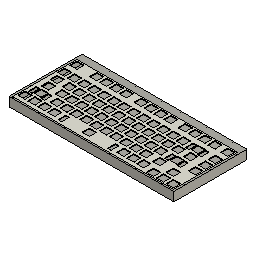
Keyboard_case (Autodesk Fusion 360 design; units mm, degrees)
part number: 2026-03-22-16-39-54-698
Autodesk Fusion 360 part; units mm, degrees
note: some values were not read from the file. Set by a fixed rule: which face or edge a step refers to.
(part 1 of 2)
sketch "plate-2026-03-22T13_27_17.077Z" plane through (0, 0, 0) normal (0, 0, 1) x (1, 0, 0)
  line L0 (3.025, -2.525) -> (16.025, -2.525)
  line L1 (3.025, -16.525) -> (16.025, -16.525)
  line L2 (2.525, -3.025) -> (2.525, -16.025)
  line L3 (16.525, -3.025) -> (16.525, -16.025)
  arc A0 (3.025, -2.525) -> (2.525, -3.025) centre (3.025, -3.025) ccw
  arc A1 (16.525, -3.025) -> (16.025, -2.525) centre (16.025, -3.025) ccw
  arc A2 (2.525, -16.025) -> (3.025, -16.525) centre (3.025, -16.025) ccw
  arc A3 (16.025, -16.525) -> (16.525, -16.025) centre (16.025, -16.025) ccw
  line L4 (41.125, -2.525) -> (54.125, -2.525)
  line L5 (41.125, -16.525) -> (54.125, -16.525)
  line L6 (40.625, -3.025) -> (40.625, -16.025)
  line L7 (54.625, -3.025) -> (54.625, -16.025)
  arc A4 (41.125, -2.525) -> (40.625, -3.025) centre (41.125, -3.025) ccw
  arc A5 (54.625, -3.025) -> (54.125, -2.525) centre (54.125, -3.025) ccw
  arc A6 (40.625, -16.025) -> (41.125, -16.525) centre (41.125, -16.025) ccw
  arc A7 (54.125, -16.525) -> (54.625, -16.025) centre (54.125, -16.025) ccw
  line L8 (60.175, -2.525) -> (73.175, -2.525)
  line L9 (60.175, -16.525) -> (73.175, -16.525)
  line L10 (59.675, -3.025) -> (59.675, -16.025)
  line L11 (73.675, -3.025) -> (73.675, -16.025)
  arc A8 (60.175, -2.525) -> (59.675, -3.025) centre (60.175, -3.025) ccw
  arc A9 (73.675, -3.025) -> (73.175, -2.525) centre (73.175, -3.025) ccw
  arc A10 (59.675, -16.025) -> (60.175, -16.525) centre (60.175, -16.025) ccw
  arc A11 (73.175, -16.525) -> (73.675, -16.025) centre (73.175, -16.025) ccw
  line L12 (79.225, -2.525) -> (92.225, -2.525)
  line L13 (79.225, -16.525) -> (92.225, -16.525)
  line L14 (78.725, -3.025) -> (78.725, -16.025)
  line L15 (92.725, -3.025) -> (92.725, -16.025)
  arc A12 (79.225, -2.525) -> (78.725, -3.025) centre (79.225, -3.025) ccw
  arc A13 (92.725, -3.025) -> (92.225, -2.525) centre (92.225, -3.025) ccw
  arc A14 (78.725, -16.025) -> (79.225, -16.525) centre (79.225, -16.025) ccw
  arc A15 (92.225, -16.525) -> (92.725, -16.025) centre (92.225, -16.025) ccw
  line L16 (98.275, -2.525) -> (111.275, -2.525)
  line L17 (98.275, -16.525) -> (111.275, -16.525)
  line L18 (97.775, -3.025) -> (97.775, -16.025)
  line L19 (111.775, -3.025) -> (111.775, -16.025)
  arc A16 (98.275, -2.525) -> (97.775, -3.025) centre (98.275, -3.025) ccw
  arc A17 (111.775, -3.025) -> (111.275, -2.525) centre (111.275, -3.025) ccw
  arc A18 (97.775, -16.025) -> (98.275, -16.525) centre (98.275, -16.025) ccw
  arc A19 (111.275, -16.525) -> (111.775, -16.025) centre (111.275, -16.025) ccw
  line L20 (126.85, -2.525) -> (139.85, -2.525)
  line L21 (126.85, -16.525) -> (139.85, -16.525)
  line L22 (126.35, -3.025) -> (126.35, -16.025)
  line L23 (140.35, -3.025) -> (140.35, -16.025)
  arc A20 (126.85, -2.525) -> (126.35, -3.025) centre (126.85, -3.025) ccw
  arc A21 (140.35, -3.025) -> (139.85, -2.525) centre (139.85, -3.025) ccw
  arc A22 (126.35, -16.025) -> (126.85, -16.525) centre (126.85, -16.025) ccw
  arc A23 (139.85, -16.525) -> (140.35, -16.025) centre (139.85, -16.025) ccw
  line L24 (145.9, -2.525) -> (158.9, -2.525)
  line L25 (145.9, -16.525) -> (158.9, -16.525)
  line L26 (145.4, -3.025) -> (145.4, -16.025)
  line L27 (159.4, -3.025) -> (159.4, -16.025)
  arc A24 (145.9, -2.525) -> (145.4, -3.025) centre (145.9, -3.025) ccw
  arc A25 (159.4, -3.025) -> (158.9, -2.525) centre (158.9, -3.025) ccw
  arc A26 (145.4, -16.025) -> (145.9, -16.525) centre (145.9, -16.025) ccw
  arc A27 (158.9, -16.525) -> (159.4, -16.025) centre (158.9, -16.025) ccw
  line L28 (164.95, -2.525) -> (177.95, -2.525)
  line L29 (164.95, -16.525) -> (177.95, -16.525)
  line L30 (164.45, -3.025) -> (164.45, -16.025)
  line L31 (178.45, -3.025) -> (178.45, -16.025)
  arc A28 (164.95, -2.525) -> (164.45, -3.025) centre (164.95, -3.025) ccw
  arc A29 (178.45, -3.025) -> (177.95, -2.525) centre (177.95, -3.025) ccw
  arc A30 (164.45, -16.025) -> (164.95, -16.525) centre (164.95, -16.025) ccw
  arc A31 (177.95, -16.525) -> (178.45, -16.025) centre (177.95, -16.025) ccw
  line L32 (184, -2.525) -> (197, -2.525)
  line L33 (184, -16.525) -> (197, -16.525)
  line L34 (183.5, -3.025) -> (183.5, -16.025)
  line L35 (197.5, -3.025) -> (197.5, -16.025)
  arc A32 (184, -2.525) -> (183.5, -3.025) centre (184, -3.025) ccw
  arc A33 (197.5, -3.025) -> (197, -2.525) centre (197, -3.025) ccw
  arc A34 (183.5, -16.025) -> (184, -16.525) centre (184, -16.025) ccw
  arc A35 (197, -16.525) -> (197.5, -16.025) centre (197, -16.025) ccw
  line L36 (211.6225, -2.525) -> (224.6225, -2.525)
  line L37 (211.6225, -16.525) -> (224.6225, -16.525)
  line L38 (211.1225, -3.025) -> (211.1225, -16.025)
  line L39 (225.1225, -3.025) -> (225.1225, -16.025)
  arc A36 (211.6225, -2.525) -> (211.1225, -3.025) centre (211.6225, -3.025) ccw
  arc A37 (225.1225, -3.025) -> (224.6225, -2.525) centre (224.6225, -3.025) ccw
  arc A38 (211.1225, -16.025) -> (211.6225, -16.525) centre (211.6225, -16.025) ccw
  arc A39 (224.6225, -16.525) -> (225.1225, -16.025) centre (224.6225, -16.025) ccw
  line L40 (230.6725, -2.525) -> (243.6725, -2.525)
  line L41 (230.6725, -16.525) -> (243.6725, -16.525)
  line L42 (230.1725, -3.025) -> (230.1725, -16.025)
  line L43 (244.1725, -3.025) -> (244.1725, -16.025)
  arc A40 (230.6725, -2.525) -> (230.1725, -3.025) centre (230.6725, -3.025) ccw
  arc A41 (244.1725, -3.025) -> (243.6725, -2.525) centre (243.6725, -3.025) ccw
  arc A42 (230.1725, -16.025) -> (230.6725, -16.525) centre (230.6725, -16.025) ccw
  arc A43 (243.6725, -16.525) -> (244.1725, -16.025) centre (243.6725, -16.025) ccw
  line L44 (249.7225, -2.525) -> (262.7225, -2.525)
  line L45 (249.7225, -16.525) -> (262.7225, -16.525)
  line L46 (249.2225, -3.025) -> (249.2225, -16.025)
  line L47 (263.2225, -3.025) -> (263.2225, -16.025)
  arc A44 (249.7225, -2.525) -> (249.2225, -3.025) centre (249.7225, -3.025) ccw
  arc A45 (263.2225, -3.025) -> (262.7225, -2.525) centre (262.7225, -3.025) ccw
  arc A46 (249.2225, -16.025) -> (249.7225, -16.525) centre (249.7225, -16.025) ccw
  arc A47 (262.7225, -16.525) -> (263.2225, -16.025) centre (262.7225, -16.025) ccw
  line L48 (268.7725, -2.525) -> (281.7725, -2.525)
  line L49 (268.7725, -16.525) -> (281.7725, -16.525)
  line L50 (268.2725, -3.025) -> (268.2725, -16.025)
  line L51 (282.2725, -3.025) -> (282.2725, -16.025)
  arc A48 (268.7725, -2.525) -> (268.2725, -3.025) centre (268.7725, -3.025) ccw
  arc A49 (282.2725, -3.025) -> (281.7725, -2.525) centre (281.7725, -3.025) ccw
  arc A50 (268.2725, -16.025) -> (268.7725, -16.525) centre (268.7725, -16.025) ccw
  arc A51 (281.7725, -16.525) -> (282.2725, -16.025) centre (281.7725, -16.025) ccw
  line L52 (293.5375, -2.525) -> (306.5375, -2.525)
  line L53 (293.5375, -16.525) -> (306.5375, -16.525)
  line L54 (293.0375, -3.025) -> (293.0375, -16.025)
  line L55 (307.0375, -3.025) -> (307.0375, -16.025)
  arc A52 (293.5375, -2.525) -> (293.0375, -3.025) centre (293.5375, -3.025) ccw
  arc A53 (307.0375, -3.025) -> (306.5375, -2.525) centre (306.5375, -3.025) ccw
  arc A54 (293.0375, -16.025) -> (293.5375, -16.525) centre (293.5375, -16.025) ccw
  arc A55 (306.5375, -16.525) -> (307.0375, -16.025) centre (306.5375, -16.025) ccw
  line L56 (3.025, -26.3375) -> (16.025, -26.3375)
  line L57 (3.025, -40.3375) -> (16.025, -40.3375)
  line L58 (2.525, -26.8375) -> (2.525, -39.8375)
  line L59 (16.525, -26.8375) -> (16.525, -39.8375)
  arc A56 (3.025, -26.3375) -> (2.525, -26.8375) centre (3.025, -26.8375) ccw
  arc A57 (16.525, -26.8375) -> (16.025, -26.3375) centre (16.025, -26.8375) ccw
  arc A58 (2.525, -39.8375) -> (3.025, -40.3375) centre (3.025, -39.8375) ccw
  arc A59 (16.025, -40.3375) -> (16.525, -39.8375) centre (16.025, -39.8375) ccw
  line L60 (22.075, -26.3375) -> (35.075, -26.3375)
  line L61 (22.075, -40.3375) -> (35.075, -40.3375)
  line L62 (21.575, -26.8375) -> (21.575, -39.8375)
  line L63 (35.575, -26.8375) -> (35.575, -39.8375)
  arc A60 (22.075, -26.3375) -> (21.575, -26.8375) centre (22.075, -26.8375) ccw
  arc A61 (35.575, -26.8375) -> (35.075, -26.3375) centre (35.075, -26.8375) ccw
  arc A62 (21.575, -39.8375) -> (22.075, -40.3375) centre (22.075, -39.8375) ccw
  arc A63 (35.075, -40.3375) -> (35.575, -39.8375) centre (35.075, -39.8375) ccw
  line L64 (41.125, -26.3375) -> (54.125, -26.3375)
  line L65 (41.125, -40.3375) -> (54.125, -40.3375)
  line L66 (40.625, -26.8375) -> (40.625, -39.8375)
  line L67 (54.625, -26.8375) -> (54.625, -39.8375)
  arc A64 (41.125, -26.3375) -> (40.625, -26.8375) centre (41.125, -26.8375) ccw
  arc A65 (54.625, -26.8375) -> (54.125, -26.3375) centre (54.125, -26.8375) ccw
  arc A66 (40.625, -39.8375) -> (41.125, -40.3375) centre (41.125, -39.8375) ccw
  arc A67 (54.125, -40.3375) -> (54.625, -39.8375) centre (54.125, -39.8375) ccw
  line L68 (60.175, -26.3375) -> (73.175, -26.3375)
  line L69 (60.175, -40.3375) -> (73.175, -40.3375)
  line L70 (59.675, -26.8375) -> (59.675, -39.8375)
  line L71 (73.675, -26.8375) -> (73.675, -39.8375)
  arc A68 (60.175, -26.3375) -> (59.675, -26.8375) centre (60.175, -26.8375) ccw
  arc A69 (73.675, -26.8375) -> (73.175, -26.3375) centre (73.175, -26.8375) ccw
  arc A70 (59.675, -39.8375) -> (60.175, -40.3375) centre (60.175, -39.8375) ccw
  arc A71 (73.175, -40.3375) -> (73.675, -39.8375) centre (73.175, -39.8375) ccw
  line L72 (79.225, -26.3375) -> (92.225, -26.3375)
  line L73 (79.225, -40.3375) -> (92.225, -40.3375)
  line L74 (78.725, -26.8375) -> (78.725, -39.8375)
  line L75 (92.725, -26.8375) -> (92.725, -39.8375)
  arc A72 (79.225, -26.3375) -> (78.725, -26.8375) centre (79.225, -26.8375) ccw
  arc A73 (92.725, -26.8375) -> (92.225, -26.3375) centre (92.225, -26.8375) ccw
  arc A74 (78.725, -39.8375) -> (79.225, -40.3375) centre (79.225, -39.8375) ccw
  arc A75 (92.225, -40.3375) -> (92.725, -39.8375) centre (92.225, -39.8375) ccw
  line L76 (98.275, -26.3375) -> (111.275, -26.3375)
  line L77 (98.275, -40.3375) -> (111.275, -40.3375)
  line L78 (97.775, -26.8375) -> (97.775, -39.8375)
  line L79 (111.775, -26.8375) -> (111.775, -39.8375)
  arc A76 (98.275, -26.3375) -> (97.775, -26.8375) centre (98.275, -26.8375) ccw
  arc A77 (111.775, -26.8375) -> (111.275, -26.3375) centre (111.275, -26.8375) ccw
  arc A78 (97.775, -39.8375) -> (98.275, -40.3375) centre (98.275, -39.8375) ccw
  arc A79 (111.275, -40.3375) -> (111.775, -39.8375) centre (111.275, -39.8375) ccw
  line L80 (117.325, -26.3375) -> (130.325, -26.3375)
  line L81 (117.325, -40.3375) -> (130.325, -40.3375)
  line L82 (116.825, -26.8375) -> (116.825, -39.8375)
  line L83 (130.825, -26.8375) -> (130.825, -39.8375)
  arc A80 (117.325, -26.3375) -> (116.825, -26.8375) centre (117.325, -26.8375) ccw
  arc A81 (130.825, -26.8375) -> (130.325, -26.3375) centre (130.325, -26.8375) ccw
  arc A82 (116.825, -39.8375) -> (117.325, -40.3375) centre (117.325, -39.8375) ccw
  arc A83 (130.325, -40.3375) -> (130.825, -39.8375) centre (130.325, -39.8375) ccw
  line L84 (136.375, -26.3375) -> (149.375, -26.3375)
  line L85 (136.375, -40.3375) -> (149.375, -40.3375)
  line L86 (135.875, -26.8375) -> (135.875, -39.8375)
  line L87 (149.875, -26.8375) -> (149.875, -39.8375)
  arc A84 (136.375, -26.3375) -> (135.875, -26.8375) centre (136.375, -26.8375) ccw
  arc A85 (149.875, -26.8375) -> (149.375, -26.3375) centre (149.375, -26.8375) ccw
  arc A86 (135.875, -39.8375) -> (136.375, -40.3375) centre (136.375, -39.8375) ccw
  arc A87 (149.375, -40.3375) -> (149.875, -39.8375) centre (149.375, -39.8375) ccw
  line L88 (155.425, -26.3375) -> (168.425, -26.3375)
  line L89 (155.425, -40.3375) -> (168.425, -40.3375)
  line L90 (154.925, -26.8375) -> (154.925, -39.8375)
  line L91 (168.925, -26.8375) -> (168.925, -39.8375)
  arc A88 (155.425, -26.3375) -> (154.925, -26.8375) centre (155.425, -26.8375) ccw
  arc A89 (168.925, -26.8375) -> (168.425, -26.3375) centre (168.425, -26.8375) ccw
  arc A90 (154.925, -39.8375) -> (155.425, -40.3375) centre (155.425, -39.8375) ccw
  arc A91 (168.425, -40.3375) -> (168.925, -39.8375) centre (168.425, -39.8375) ccw
  line L92 (174.475, -26.3375) -> (187.475, -26.3375)
  line L93 (174.475, -40.3375) -> (187.475, -40.3375)
  line L94 (173.975, -26.8375) -> (173.975, -39.8375)
  line L95 (187.975, -26.8375) -> (187.975, -39.8375)
  arc A92 (174.475, -26.3375) -> (173.975, -26.8375) centre (174.475, -26.8375) ccw
  arc A93 (187.975, -26.8375) -> (187.475, -26.3375) centre (187.475, -26.8375) ccw
  arc A94 (173.975, -39.8375) -> (174.475, -40.3375) centre (174.475, -39.8375) ccw
  arc A95 (187.475, -40.3375) -> (187.975, -39.8375) centre (187.475, -39.8375) ccw
  line L96 (193.525, -26.3375) -> (206.525, -26.3375)
  line L97 (193.525, -40.3375) -> (206.525, -40.3375)
  line L98 (193.025, -26.8375) -> (193.025, -39.8375)
  line L99 (207.025, -26.8375) -> (207.025, -39.8375)
  arc A96 (193.525, -26.3375) -> (193.025, -26.8375) centre (193.525, -26.8375) ccw
  arc A97 (207.025, -26.8375) -> (206.525, -26.3375) centre (206.525, -26.8375) ccw
  arc A98 (193.025, -39.8375) -> (193.525, -40.3375) centre (193.525, -39.8375) ccw
  arc A99 (206.525, -40.3375) -> (207.025, -39.8375) centre (206.525, -39.8375) ccw
  line L100 (212.575, -26.3375) -> (225.575, -26.3375)
  line L101 (212.575, -40.3375) -> (225.575, -40.3375)
  line L102 (212.075, -26.8375) -> (212.075, -39.8375)
  line L103 (226.075, -26.8375) -> (226.075, -39.8375)
  arc A100 (212.575, -26.3375) -> (212.075, -26.8375) centre (212.575, -26.8375) ccw
  arc A101 (226.075, -26.8375) -> (225.575, -26.3375) centre (225.575, -26.8375) ccw
  arc A102 (212.075, -39.8375) -> (212.575, -40.3375) centre (212.575, -39.8375) ccw
  arc A103 (225.575, -40.3375) -> (226.075, -39.8375) centre (225.575, -39.8375) ccw
  line L104 (231.625, -26.3375) -> (244.625, -26.3375)
  line L105 (231.625, -40.3375) -> (244.625, -40.3375)
  line L106 (231.125, -26.8375) -> (231.125, -39.8375)
  line L107 (245.125, -26.8375) -> (245.125, -39.8375)
  arc A104 (231.625, -26.3375) -> (231.125, -26.8375) centre (231.625, -26.8375) ccw
  arc A105 (245.125, -26.8375) -> (244.625, -26.3375) centre (244.625, -26.8375) ccw
  arc A106 (231.125, -39.8375) -> (231.625, -40.3375) centre (231.625, -39.8375) ccw
  arc A107 (244.625, -40.3375) -> (245.125, -39.8375) centre (244.625, -39.8375) ccw
  line L108 (260.2, -26.3375) -> (273.2, -26.3375)
  line L109 (260.2, -40.3375) -> (273.2, -40.3375)
  line L110 (259.7, -26.8375) -> (259.7, -39.8375)
  line L111 (273.7, -26.8375) -> (273.7, -39.8375)
  arc A108 (260.2, -26.3375) -> (259.7, -26.8375) centre (260.2, -26.8375) ccw
  arc A109 (273.7, -26.8375) -> (273.2, -26.3375) centre (273.2, -26.8375) ccw
  arc A110 (259.7, -39.8375) -> (260.2, -40.3375) centre (260.2, -39.8375) ccw
  arc A111 (273.2, -40.3375) -> (273.7, -39.8375) centre (273.2, -39.8375) ccw
  line L112 (251.762, -27.3375) -> (257.762, -27.3375)
  line L113 (251.762, -42.3375) -> (257.762, -42.3375)
  line L114 (251.262, -27.8375) -> (251.262, -41.8375)
  line L115 (258.262, -27.8375) -> (258.262, -41.8375)
  arc A112 (251.762, -27.3375) -> (251.262, -27.8375) centre (251.762, -27.8375) ccw
  arc A113 (258.262, -27.8375) -> (257.762, -27.3375) centre (257.762, -27.8375) ccw
  arc A114 (251.262, -41.8375) -> (251.762, -42.3375) centre (251.762, -41.8375) ccw
  arc A115 (257.762, -42.3375) -> (258.262, -41.8375) centre (257.762, -41.8375) ccw
  line L116 (275.638, -27.3375) -> (281.638, -27.3375)
  line L117 (275.638, -42.3375) -> (281.638, -42.3375)
  line L118 (275.138, -27.8375) -> (275.138, -41.8375)
  line L119 (282.138, -27.8375) -> (282.138, -41.8375)
  arc A116 (275.638, -27.3375) -> (275.138, -27.8375) centre (275.638, -27.8375) ccw
  arc A117 (282.138, -27.8375) -> (281.638, -27.3375) centre (281.638, -27.8375) ccw
  arc A118 (275.138, -41.8375) -> (275.638, -42.3375) centre (275.638, -41.8375) ccw
  arc A119 (281.638, -42.3375) -> (282.138, -41.8375) centre (281.638, -41.8375) ccw
  line L120 (293.5375, -26.3375) -> (306.5375, -26.3375)
  line L121 (293.5375, -40.3375) -> (306.5375, -40.3375)
  line L122 (293.0375, -26.8375) -> (293.0375, -39.8375)
  line L123 (307.0375, -26.8375) -> (307.0375, -39.8375)
  arc A120 (293.5375, -26.3375) -> (293.0375, -26.8375) centre (293.5375, -26.8375) ccw
  arc A121 (307.0375, -26.8375) -> (306.5375, -26.3375) centre (306.5375, -26.8375) ccw
  arc A122 (293.0375, -39.8375) -> (293.5375, -40.3375) centre (293.5375, -39.8375) ccw
  arc A123 (306.5375, -40.3375) -> (307.0375, -39.8375) centre (306.5375, -39.8375) ccw
  line L124 (7.7875, -45.3875) -> (20.7875, -45.3875)
  line L125 (7.7875, -59.3875) -> (20.7875, -59.3875)
  line L126 (7.2875, -45.8875) -> (7.2875, -58.8875)
  line L127 (21.2875, -45.8875) -> (21.2875, -58.8875)
  arc A124 (7.7875, -45.3875) -> (7.2875, -45.8875) centre (7.7875, -45.8875) ccw
  arc A125 (21.2875, -45.8875) -> (20.7875, -45.3875) centre (20.7875, -45.8875) ccw
  arc A126 (7.2875, -58.8875) -> (7.7875, -59.3875) centre (7.7875, -58.8875) ccw
  arc A127 (20.7875, -59.3875) -> (21.2875, -58.8875) centre (20.7875, -58.8875) ccw
  line L128 (31.6, -45.3875) -> (44.6, -45.3875)
  line L129 (31.6, -59.3875) -> (44.6, -59.3875)
  line L130 (31.1, -45.8875) -> (31.1, -58.8875)
  line L131 (45.1, -45.8875) -> (45.1, -58.8875)
  arc A128 (31.6, -45.3875) -> (31.1, -45.8875) centre (31.6, -45.8875) ccw
  arc A129 (45.1, -45.8875) -> (44.6, -45.3875) centre (44.6, -45.8875) ccw
  arc A130 (31.1, -58.8875) -> (31.6, -59.3875) centre (31.6, -58.8875) ccw
  arc A131 (44.6, -59.3875) -> (45.1, -58.8875) centre (44.6, -58.8875) ccw
  line L132 (50.65, -45.3875) -> (63.65, -45.3875)
  line L133 (50.65, -59.3875) -> (63.65, -59.3875)
  line L134 (50.15, -45.8875) -> (50.15, -58.8875)
  line L135 (64.15, -45.8875) -> (64.15, -58.8875)
  arc A132 (50.65, -45.3875) -> (50.15, -45.8875) centre (50.65, -45.8875) ccw
  arc A133 (64.15, -45.8875) -> (63.65, -45.3875) centre (63.65, -45.8875) ccw
  arc A134 (50.15, -58.8875) -> (50.65, -59.3875) centre (50.65, -58.8875) ccw
  arc A135 (63.65, -59.3875) -> (64.15, -58.8875) centre (63.65, -58.8875) ccw
  line L136 (69.7, -45.3875) -> (82.7, -45.3875)
  line L137 (69.7, -59.3875) -> (82.7, -59.3875)
  line L138 (69.2, -45.8875) -> (69.2, -58.8875)
  line L139 (83.2, -45.8875) -> (83.2, -58.8875)
  arc A136 (69.7, -45.3875) -> (69.2, -45.8875) centre (69.7, -45.8875) ccw
  arc A137 (83.2, -45.8875) -> (82.7, -45.3875) centre (82.7, -45.8875) ccw
  arc A138 (69.2, -58.8875) -> (69.7, -59.3875) centre (69.7, -58.8875) ccw
  arc A139 (82.7, -59.3875) -> (83.2, -58.8875) centre (82.7, -58.8875) ccw
  line L140 (88.75, -45.3875) -> (101.75, -45.3875)
  line L141 (88.75, -59.3875) -> (101.75, -59.3875)
  line L142 (88.25, -45.8875) -> (88.25, -58.8875)
  line L143 (102.25, -45.8875) -> (102.25, -58.8875)
  arc A140 (88.75, -45.3875) -> (88.25, -45.8875) centre (88.75, -45.8875) ccw
  arc A141 (102.25, -45.8875) -> (101.75, -45.3875) centre (101.75, -45.8875) ccw
  arc A142 (88.25, -58.8875) -> (88.75, -59.3875) centre (88.75, -58.8875) ccw
  arc A143 (101.75, -59.3875) -> (102.25, -58.8875) centre (101.75, -58.8875) ccw
  line L144 (107.8, -45.3875) -> (120.8, -45.3875)
  line L145 (107.8, -59.3875) -> (120.8, -59.3875)
  line L146 (107.3, -45.8875) -> (107.3, -58.8875)
  line L147 (121.3, -45.8875) -> (121.3, -58.8875)
  arc A144 (107.8, -45.3875) -> (107.3, -45.8875) centre (107.8, -45.8875) ccw
  arc A145 (121.3, -45.8875) -> (120.8, -45.3875) centre (120.8, -45.8875) ccw
  arc A146 (107.3, -58.8875) -> (107.8, -59.3875) centre (107.8, -58.8875) ccw
  arc A147 (120.8, -59.3875) -> (121.3, -58.8875) centre (120.8, -58.8875) ccw
  line L148 (126.85, -45.3875) -> (139.85, -45.3875)
  line L149 (126.85, -59.3875) -> (139.85, -59.3875)
  line L150 (126.35, -45.8875) -> (126.35, -58.8875)
  line L151 (140.35, -45.8875) -> (140.35, -58.8875)
  arc A148 (126.85, -45.3875) -> (126.35, -45.8875) centre (126.85, -45.8875) ccw
  arc A149 (140.35, -45.8875) -> (139.85, -45.3875) centre (139.85, -45.8875) ccw
  arc A150 (126.35, -58.8875) -> (126.85, -59.3875) centre (126.85, -58.8875) ccw
  arc A151 (139.85, -59.3875) -> (140.35, -58.8875) centre (139.85, -58.8875) ccw
  line L152 (145.9, -45.3875) -> (158.9, -45.3875)
  line L153 (145.9, -59.3875) -> (158.9, -59.3875)
  line L154 (145.4, -45.8875) -> (145.4, -58.8875)
  line L155 (159.4, -45.8875) -> (159.4, -58.8875)
  arc A152 (145.9, -45.3875) -> (145.4, -45.8875) centre (145.9, -45.8875) ccw
  arc A153 (159.4, -45.8875) -> (158.9, -45.3875) centre (158.9, -45.8875) ccw
  arc A154 (145.4, -58.8875) -> (145.9, -59.3875) centre (145.9, -58.8875) ccw
  arc A155 (158.9, -59.3875) -> (159.4, -58.8875) centre (158.9, -58.8875) ccw
  line L156 (164.95, -45.3875) -> (177.95, -45.3875)
  line L157 (164.95, -59.3875) -> (177.95, -59.3875)
  line L158 (164.45, -45.8875) -> (164.45, -58.8875)
  line L159 (178.45, -45.8875) -> (178.45, -58.8875)
  arc A156 (164.95, -45.3875) -> (164.45, -45.8875) centre (164.95, -45.8875) ccw
  arc A157 (178.45, -45.8875) -> (177.95, -45.3875) centre (177.95, -45.8875) ccw
  arc A158 (164.45, -58.8875) -> (164.95, -59.3875) centre (164.95, -58.8875) ccw
  arc A159 (177.95, -59.3875) -> (178.45, -58.8875) centre (177.95, -58.8875) ccw
  line L160 (184, -45.3875) -> (197, -45.3875)
  line L161 (184, -59.3875) -> (197, -59.3875)
  line L162 (183.5, -45.8875) -> (183.5, -58.8875)
  line L163 (197.5, -45.8875) -> (197.5, -58.8875)
  arc A160 (184, -45.3875) -> (183.5, -45.8875) centre (184, -45.8875) ccw
  arc A161 (197.5, -45.8875) -> (197, -45.3875) centre (197, -45.8875) ccw
  arc A162 (183.5, -58.8875) -> (184, -59.3875) centre (184, -58.8875) ccw
  arc A163 (197, -59.3875) -> (197.5, -58.8875) centre (197, -58.8875) ccw
  line L164 (203.05, -45.3875) -> (216.05, -45.3875)
  line L165 (203.05, -59.3875) -> (216.05, -59.3875)
  line L166 (202.55, -45.8875) -> (202.55, -58.8875)
  line L167 (216.55, -45.8875) -> (216.55, -58.8875)
  arc A164 (203.05, -45.3875) -> (202.55, -45.8875) centre (203.05, -45.8875) ccw
  arc A165 (216.55, -45.8875) -> (216.05, -45.3875) centre (216.05, -45.8875) ccw
  arc A166 (202.55, -58.8875) -> (203.05, -59.3875) centre (203.05, -58.8875) ccw
  arc A167 (216.05, -59.3875) -> (216.55, -58.8875) centre (216.05, -58.8875) ccw
  line L168 (222.1, -45.3875) -> (235.1, -45.3875)
  line L169 (222.1, -59.3875) -> (235.1, -59.3875)
  line L170 (221.6, -45.8875) -> (221.6, -58.8875)
  line L171 (235.6, -45.8875) -> (235.6, -58.8875)
  arc A168 (222.1, -45.3875) -> (221.6, -45.8875) centre (222.1, -45.8875) ccw
  arc A169 (235.6, -45.8875) -> (235.1, -45.3875) centre (235.1, -45.8875) ccw
  arc A170 (221.6, -58.8875) -> (222.1, -59.3875) centre (222.1, -58.8875) ccw
  arc A171 (235.1, -59.3875) -> (235.6, -58.8875) centre (235.1, -58.8875) ccw
  line L172 (241.15, -45.3875) -> (254.15, -45.3875)
  line L173 (241.15, -59.3875) -> (254.15, -59.3875)
  line L174 (240.65, -45.8875) -> (240.65, -58.8875)
  line L175 (254.65, -45.8875) -> (254.65, -58.8875)
  arc A172 (241.15, -45.3875) -> (240.65, -45.8875) centre (241.15, -45.8875) ccw
  arc A173 (254.65, -45.8875) -> (254.15, -45.3875) centre (254.15, -45.8875) ccw
  arc A174 (240.65, -58.8875) -> (241.15, -59.3875) centre (241.15, -58.8875) ccw
  arc A175 (254.15, -59.3875) -> (254.65, -58.8875) centre (254.15, -58.8875) ccw
  line L176 (264.9625, -45.3875) -> (277.9625, -45.3875)
  line L177 (264.9625, -59.3875) -> (277.9625, -59.3875)
  line L178 (264.4625, -45.8875) -> (264.4625, -58.8875)
  line L179 (278.4625, -45.8875) -> (278.4625, -58.8875)
  arc A176 (264.9625, -45.3875) -> (264.4625, -45.8875) centre (264.9625, -45.8875) ccw
  arc A177 (278.4625, -45.8875) -> (277.9625, -45.3875) centre (277.9625, -45.8875) ccw
  arc A178 (264.4625, -58.8875) -> (264.9625, -59.3875) centre (264.9625, -58.8875) ccw
  arc A179 (277.9625, -59.3875) -> (278.4625, -58.8875) centre (277.9625, -58.8875) ccw
  line L180 (293.5375, -45.3875) -> (306.5375, -45.3875)
  line L181 (293.5375, -59.3875) -> (306.5375, -59.3875)
  line L182 (293.0375, -45.8875) -> (293.0375, -58.8875)
  line L183 (307.0375, -45.8875) -> (307.0375, -58.8875)
  arc A180 (293.5375, -45.3875) -> (293.0375, -45.8875) centre (293.5375, -45.8875) ccw
  arc A181 (307.0375, -45.8875) -> (306.5375, -45.3875) centre (306.5375, -45.8875) ccw
  arc A182 (293.0375, -58.8875) -> (293.5375, -59.3875) centre (293.5375, -58.8875) ccw
  arc A183 (306.5375, -59.3875) -> (307.0375, -58.8875) centre (306.5375, -58.8875) ccw
  line L184 (10.1687, -64.4375) -> (23.1687, -64.4375)
  line L185 (10.1687, -78.4375) -> (23.1687, -78.4375)
  line L186 (9.6687, -64.9375) -> (9.6687, -77.9375)
  line L187 (23.6687, -64.9375) -> (23.6687, -77.9375)
  arc A184 (10.1687, -64.4375) -> (9.6688, -64.9375) centre (10.1687, -64.9375) ccw
  arc A185 (23.6687, -64.9375) -> (23.1687, -64.4375) centre (23.1687, -64.9375) ccw
  arc A186 (9.6687, -77.9375) -> (10.1687, -78.4375) centre (10.1687, -77.9375) ccw
  arc A187 (23.1687, -78.4375) -> (23.6687, -77.9375) centre (23.1687, -77.9375) ccw
  line L188 (36.3625, -64.4375) -> (49.3625, -64.4375)
  line L189 (36.3625, -78.4375) -> (49.3625, -78.4375)
  line L190 (35.8625, -64.9375) -> (35.8625, -77.9375)
  line L191 (49.8625, -64.9375) -> (49.8625, -77.9375)
  arc A188 (36.3625, -64.4375) -> (35.8625, -64.9375) centre (36.3625, -64.9375) ccw
  arc A189 (49.8625, -64.9375) -> (49.3625, -64.4375) centre (49.3625, -64.9375) ccw
  arc A190 (35.8625, -77.9375) -> (36.3625, -78.4375) centre (36.3625, -77.9375) ccw
  arc A191 (49.3625, -78.4375) -> (49.8625, -77.9375) centre (49.3625, -77.9375) ccw
  line L192 (55.4125, -64.4375) -> (68.4125, -64.4375)
  line L193 (55.4125, -78.4375) -> (68.4125, -78.4375)
  line L194 (54.9125, -64.9375) -> (54.9125, -77.9375)
  line L195 (68.9125, -64.9375) -> (68.9125, -77.9375)
  arc A192 (55.4125, -64.4375) -> (54.9125, -64.9375) centre (55.4125, -64.9375) ccw
  arc A193 (68.9125, -64.9375) -> (68.4125, -64.4375) centre (68.4125, -64.9375) ccw
  arc A194 (54.9125, -77.9375) -> (55.4125, -78.4375) centre (55.4125, -77.9375) ccw
  arc A195 (68.4125, -78.4375) -> (68.9125, -77.9375) centre (68.4125, -77.9375) ccw
  line L196 (74.4625, -64.4375) -> (87.4625, -64.4375)
  line L197 (74.4625, -78.4375) -> (87.4625, -78.4375)
  line L198 (73.9625, -64.9375) -> (73.9625, -77.9375)
  line L199 (87.9625, -64.9375) -> (87.9625, -77.9375)
  arc A196 (74.4625, -64.4375) -> (73.9625, -64.9375) centre (74.4625, -64.9375) ccw
  arc A197 (87.9625, -64.9375) -> (87.4625, -64.4375) centre (87.4625, -64.9375) ccw
  arc A198 (73.9625, -77.9375) -> (74.4625, -78.4375) centre (74.4625, -77.9375) ccw
  arc A199 (87.4625, -78.4375) -> (87.9625, -77.9375) centre (87.4625, -77.9375) ccw
  line L200 (93.5125, -64.4375) -> (106.5125, -64.4375)
  line L201 (93.5125, -78.4375) -> (106.5125, -78.4375)
  line L202 (93.0125, -64.9375) -> (93.0125, -77.9375)
  line L203 (107.0125, -64.9375) -> (107.0125, -77.9375)
  arc A200 (93.5125, -64.4375) -> (93.0125, -64.9375) centre (93.5125, -64.9375) ccw
  arc A201 (107.0125, -64.9375) -> (106.5125, -64.4375) centre (106.5125, -64.9375) ccw
  arc A202 (93.0125, -77.9375) -> (93.5125, -78.4375) centre (93.5125, -77.9375) ccw
  arc A203 (106.5125, -78.4375) -> (107.0125, -77.9375) centre (106.5125, -77.9375) ccw
  line L204 (112.5625, -64.4375) -> (125.5625, -64.4375)
  line L205 (112.5625, -78.4375) -> (125.5625, -78.4375)
  line L206 (112.0625, -64.9375) -> (112.0625, -77.9375)
  line L207 (126.0625, -64.9375) -> (126.0625, -77.9375)
  arc A204 (112.5625, -64.4375) -> (112.0625, -64.9375) centre (112.5625, -64.9375) ccw
  arc A205 (126.0625, -64.9375) -> (125.5625, -64.4375) centre (125.5625, -64.9375) ccw
  arc A206 (112.0625, -77.9375) -> (112.5625, -78.4375) centre (112.5625, -77.9375) ccw
  arc A207 (125.5625, -78.4375) -> (126.0625, -77.9375) centre (125.5625, -77.9375) ccw
  line L208 (131.6125, -64.4375) -> (144.6125, -64.4375)
  line L209 (131.6125, -78.4375) -> (144.6125, -78.4375)
  line L210 (131.1125, -64.9375) -> (131.1125, -77.9375)
  line L211 (145.1125, -64.9375) -> (145.1125, -77.9375)
  arc A208 (131.6125, -64.4375) -> (131.1125, -64.9375) centre (131.6125, -64.9375) ccw
  arc A209 (145.1125, -64.9375) -> (144.6125, -64.4375) centre (144.6125, -64.9375) ccw
  arc A210 (131.1125, -77.9375) -> (131.6125, -78.4375) centre (131.6125, -77.9375) ccw
  arc A211 (144.6125, -78.4375) -> (145.1125, -77.9375) centre (144.6125, -77.9375) ccw
  line L212 (150.6625, -64.4375) -> (163.6625, -64.4375)
  line L213 (150.6625, -78.4375) -> (163.6625, -78.4375)
  line L214 (150.1625, -64.9375) -> (150.1625, -77.9375)
  line L215 (164.1625, -64.9375) -> (164.1625, -77.9375)
  arc A212 (150.6625, -64.4375) -> (150.1625, -64.9375) centre (150.6625, -64.9375) ccw
  arc A213 (164.1625, -64.9375) -> (163.6625, -64.4375) centre (163.6625, -64.9375) ccw
  arc A214 (150.1625, -77.9375) -> (150.6625, -78.4375) centre (150.6625, -77.9375) ccw
  arc A215 (163.6625, -78.4375) -> (164.1625, -77.9375) centre (163.6625, -77.9375) ccw
  line L216 (169.7125, -64.4375) -> (182.7125, -64.4375)
  line L217 (169.7125, -78.4375) -> (182.7125, -78.4375)
  line L218 (169.2125, -64.9375) -> (169.2125, -77.9375)
  line L219 (183.2125, -64.9375) -> (183.2125, -77.9375)
  arc A216 (169.7125, -64.4375) -> (169.2125, -64.9375) centre (169.7125, -64.9375) ccw
  arc A217 (183.2125, -64.9375) -> (182.7125, -64.4375) centre (182.7125, -64.9375) ccw
  arc A218 (169.2125, -77.9375) -> (169.7125, -78.4375) centre (169.7125, -77.9375) ccw
  arc A219 (182.7125, -78.4375) -> (183.2125, -77.9375) centre (182.7125, -77.9375) ccw
  line L220 (188.7625, -64.4375) -> (201.7625, -64.4375)
  line L221 (188.7625, -78.4375) -> (201.7625, -78.4375)
  line L222 (188.2625, -64.9375) -> (188.2625, -77.9375)
  line L223 (202.2625, -64.9375) -> (202.2625, -77.9375)
  arc A220 (188.7625, -64.4375) -> (188.2625, -64.9375) centre (188.7625, -64.9375) ccw
  arc A221 (202.2625, -64.9375) -> (201.7625, -64.4375) centre (201.7625, -64.9375) ccw
  arc A222 (188.2625, -77.9375) -> (188.7625, -78.4375) centre (188.7625, -77.9375) ccw
  arc A223 (201.7625, -78.4375) -> (202.2625, -77.9375) centre (201.7625, -77.9375) ccw
  line L224 (207.8125, -64.4375) -> (220.8125, -64.4375)
  line L225 (207.8125, -78.4375) -> (220.8125, -78.4375)
  line L226 (207.3125, -64.9375) -> (207.3125, -77.9375)
  line L227 (221.3125, -64.9375) -> (221.3125, -77.9375)
  arc A224 (207.8125, -64.4375) -> (207.3125, -64.9375) centre (207.8125, -64.9375) ccw
  arc A225 (221.3125, -64.9375) -> (220.8125, -64.4375) centre (220.8125, -64.9375) ccw
  arc A226 (207.3125, -77.9375) -> (207.8125, -78.4375) centre (207.8125, -77.9375) ccw
  arc A227 (220.8125, -78.4375) -> (221.3125, -77.9375) centre (220.8125, -77.9375) ccw
  line L228 (226.8625, -64.4375) -> (239.8625, -64.4375)
  line L229 (226.8625, -78.4375) -> (239.8625, -78.4375)
  line L230 (226.3625, -64.9375) -> (226.3625, -77.9375)
  line L231 (240.3625, -64.9375) -> (240.3625, -77.9375)
  arc A228 (226.8625, -64.4375) -> (226.3625, -64.9375) centre (226.8625, -64.9375) ccw
  arc A229 (240.3625, -64.9375) -> (239.8625, -64.4375) centre (239.8625, -64.9375) ccw
  arc A230 (226.3625, -77.9375) -> (226.8625, -78.4375) centre (226.8625, -77.9375) ccw
  arc A231 (239.8625, -78.4375) -> (240.3625, -77.9375) centre (239.8625, -77.9375) ccw
  line L232 (257.8188, -64.4375) -> (270.8188, -64.4375)
  line L233 (257.8188, -78.4375) -> (270.8188, -78.4375)
  line L234 (257.3188, -64.9375) -> (257.3188, -77.9375)
  line L235 (271.3188, -64.9375) -> (271.3188, -77.9375)
  arc A232 (257.8188, -64.4375) -> (257.3188, -64.9375) centre (257.8188, -64.9375) ccw
  arc A233 (271.3188, -64.9375) -> (270.8188, -64.4375) centre (270.8188, -64.9375) ccw
  arc A234 (257.3188, -77.9375) -> (257.8188, -78.4375) centre (257.8188, -77.9375) ccw
  arc A235 (270.8188, -78.4375) -> (271.3188, -77.9375) centre (270.8188, -77.9375) ccw
  line L236 (249.3808, -65.4375) -> (255.3808, -65.4375)
  line L237 (249.3808, -80.4375) -> (255.3808, -80.4375)
  line L238 (248.8808, -65.9375) -> (248.8808, -79.9375)
  line L239 (255.8808, -65.9375) -> (255.8808, -79.9375)
  arc A236 (249.3808, -65.4375) -> (248.8808, -65.9375) centre (249.3808, -65.9375) ccw
  arc A237 (255.8808, -65.9375) -> (255.3808, -65.4375) centre (255.3808, -65.9375) ccw
  arc A238 (248.8808, -79.9375) -> (249.3808, -80.4375) centre (249.3808, -79.9375) ccw
  arc A239 (255.3808, -80.4375) -> (255.8808, -79.9375) centre (255.3808, -79.9375) ccw
  line L240 (273.2568, -65.4375) -> (279.2568, -65.4375)
  line L241 (273.2568, -80.4375) -> (279.2568, -80.4375)
  line L242 (272.7568, -65.9375) -> (272.7568, -79.9375)
  line L243 (279.7568, -65.9375) -> (279.7568, -79.9375)
  arc A240 (273.2568, -65.4375) -> (272.7568, -65.9375) centre (273.2568, -65.9375) ccw
  arc A241 (279.7568, -65.9375) -> (279.2568, -65.4375) centre (279.2568, -65.9375) ccw
  arc A242 (272.7568, -79.9375) -> (273.2568, -80.4375) centre (273.2568, -79.9375) ccw
  arc A243 (279.2568, -80.4375) -> (279.7568, -79.9375) centre (279.2568, -79.9375) ccw
  line L244 (293.5375, -64.4375) -> (306.5375, -64.4375)
  line L245 (293.5375, -78.4375) -> (306.5375, -78.4375)
  line L246 (293.0375, -64.9375) -> (293.0375, -77.9375)
  line L247 (307.0375, -64.9375) -> (307.0375, -77.9375)
  arc A244 (293.5375, -64.4375) -> (293.0375, -64.9375) centre (293.5375, -64.9375) ccw
  arc A245 (307.0375, -64.9375) -> (306.5375, -64.4375) centre (306.5375, -64.9375) ccw
  arc A246 (293.0375, -77.9375) -> (293.5375, -78.4375) centre (293.5375, -77.9375) ccw
  arc A247 (306.5375, -78.4375) -> (307.0375, -77.9375) centre (306.5375, -77.9375) ccw
  line L248 (14.9313, -83.4875) -> (27.9312, -83.4875)
  line L249 (14.9313, -97.4875) -> (27.9312, -97.4875)
  line L250 (14.4313, -83.9875) -> (14.4313, -96.9875)
  line L251 (28.4313, -83.9875) -> (28.4313, -96.9875)
  arc A248 (14.9313, -83.4875) -> (14.4313, -83.9875) centre (14.9313, -83.9875) ccw
  arc A249 (28.4313, -83.9875) -> (27.9312, -83.4875) centre (27.9312, -83.9875) ccw
  arc A250 (14.4313, -96.9875) -> (14.9313, -97.4875) centre (14.9313, -96.9875) ccw
  arc A251 (27.9312, -97.4875) -> (28.4313, -96.9875) centre (27.9312, -96.9875) ccw
  line L252 (6.4933, -84.4875) -> (12.4932, -84.4875)
  line L253 (6.4933, -99.4875) -> (12.4932, -99.4875)
  line L254 (5.9932, -84.9875) -> (5.9932, -98.9875)
  line L255 (12.9932, -84.9875) -> (12.9932, -98.9875)
  arc A252 (6.4933, -84.4875) -> (5.9933, -84.9875) centre (6.4933, -84.9875) ccw
  arc A253 (12.9932, -84.9875) -> (12.4932, -84.4875) centre (12.4932, -84.9875) ccw
  arc A254 (5.9932, -98.9875) -> (6.4933, -99.4875) centre (6.4933, -98.9875) ccw
  arc A255 (12.4932, -99.4875) -> (12.9933, -98.9875) centre (12.4932, -98.9875) ccw
  line L256 (30.3693, -84.4875) -> (36.3693, -84.4875)
  line L257 (30.3693, -99.4875) -> (36.3693, -99.4875)
  line L258 (29.8693, -84.9875) -> (29.8693, -98.9875)
  line L259 (36.8693, -84.9875) -> (36.8693, -98.9875)
  arc A256 (30.3693, -84.4875) -> (29.8693, -84.9875) centre (30.3693, -84.9875) ccw
  arc A257 (36.8693, -84.9875) -> (36.3693, -84.4875) centre (36.3693, -84.9875) ccw
  arc A258 (29.8693, -98.9875) -> (30.3693, -99.4875) centre (30.3693, -98.9875) ccw
  arc A259 (36.3693, -99.4875) -> (36.8693, -98.9875) centre (36.3693, -98.9875) ccw
  line L260 (45.8875, -83.4875) -> (58.8875, -83.4875)
  line L261 (45.8875, -97.4875) -> (58.8875, -97.4875)
  line L262 (45.3875, -83.9875) -> (45.3875, -96.9875)
  line L263 (59.3875, -83.9875) -> (59.3875, -96.9875)
  arc A260 (45.8875, -83.4875) -> (45.3875, -83.9875) centre (45.8875, -83.9875) ccw
  arc A261 (59.3875, -83.9875) -> (58.8875, -83.4875) centre (58.8875, -83.9875) ccw
  arc A262 (45.3875, -96.9875) -> (45.8875, -97.4875) centre (45.8875, -96.9875) ccw
  arc A263 (58.8875, -97.4875) -> (59.3875, -96.9875) centre (58.8875, -96.9875) ccw
  line L264 (64.9375, -83.4875) -> (77.9375, -83.4875)
  line L265 (64.9375, -97.4875) -> (77.9375, -97.4875)
  line L266 (64.4375, -83.9875) -> (64.4375, -96.9875)
  line L267 (78.4375, -83.9875) -> (78.4375, -96.9875)
  arc A264 (64.9375, -83.4875) -> (64.4375, -83.9875) centre (64.9375, -83.9875) ccw
  arc A265 (78.4375, -83.9875) -> (77.9375, -83.4875) centre (77.9375, -83.9875) ccw
  arc A266 (64.4375, -96.9875) -> (64.9375, -97.4875) centre (64.9375, -96.9875) ccw
  arc A267 (77.9375, -97.4875) -> (78.4375, -96.9875) centre (77.9375, -96.9875) ccw
  line L268 (83.9875, -83.4875) -> (96.9875, -83.4875)
  line L269 (83.9875, -97.4875) -> (96.9875, -97.4875)
  line L270 (83.4875, -83.9875) -> (83.4875, -96.9875)
  line L271 (97.4875, -83.9875) -> (97.4875, -96.9875)
  arc A268 (83.9875, -83.4875) -> (83.4875, -83.9875) centre (83.9875, -83.9875) ccw
  arc A269 (97.4875, -83.9875) -> (96.9875, -83.4875) centre (96.9875, -83.9875) ccw
  arc A270 (83.4875, -96.9875) -> (83.9875, -97.4875) centre (83.9875, -96.9875) ccw
  arc A271 (96.9875, -97.4875) -> (97.4875, -96.9875) centre (96.9875, -96.9875) ccw
  line L272 (103.0375, -83.4875) -> (116.0375, -83.4875)
  line L273 (103.0375, -97.4875) -> (116.0375, -97.4875)
  line L274 (102.5375, -83.9875) -> (102.5375, -96.9875)
  line L275 (116.5375, -83.9875) -> (116.5375, -96.9875)
  arc A272 (103.0375, -83.4875) -> (102.5375, -83.9875) centre (103.0375, -83.9875) ccw
  arc A273 (116.5375, -83.9875) -> (116.0375, -83.4875) centre (116.0375, -83.9875) ccw
  arc A274 (102.5375, -96.9875) -> (103.0375, -97.4875) centre (103.0375, -96.9875) ccw
  arc A275 (116.0375, -97.4875) -> (116.5375, -96.9875) centre (116.0375, -96.9875) ccw
  line L276 (122.0875, -83.4875) -> (135.0875, -83.4875)
  line L277 (122.0875, -97.4875) -> (135.0875, -97.4875)
  line L278 (121.5875, -83.9875) -> (121.5875, -96.9875)
  line L279 (135.5875, -83.9875) -> (135.5875, -96.9875)
  arc A276 (122.0875, -83.4875) -> (121.5875, -83.9875) centre (122.0875, -83.9875) ccw
  arc A277 (135.5875, -83.9875) -> (135.0875, -83.4875) centre (135.0875, -83.9875) ccw
  arc A278 (121.5875, -96.9875) -> (122.0875, -97.4875) centre (122.0875, -96.9875) ccw
  arc A279 (135.0875, -97.4875) -> (135.5875, -96.9875) centre (135.0875, -96.9875) ccw
  line L280 (141.1375, -83.4875) -> (154.1375, -83.4875)
  line L281 (141.1375, -97.4875) -> (154.1375, -97.4875)
  line L282 (140.6375, -83.9875) -> (140.6375, -96.9875)
  line L283 (154.6375, -83.9875) -> (154.6375, -96.9875)
  arc A280 (141.1375, -83.4875) -> (140.6375, -83.9875) centre (141.1375, -83.9875) ccw
  arc A281 (154.6375, -83.9875) -> (154.1375, -83.4875) centre (154.1375, -83.9875) ccw
  arc A282 (140.6375, -96.9875) -> (141.1375, -97.4875) centre (141.1375, -96.9875) ccw
  arc A283 (154.1375, -97.4875) -> (154.6375, -96.9875) centre (154.1375, -96.9875) ccw
  line L284 (160.1875, -83.4875) -> (173.1875, -83.4875)
  line L285 (160.1875, -97.4875) -> (173.1875, -97.4875)
  line L286 (159.6875, -83.9875) -> (159.6875, -96.9875)
  line L287 (173.6875, -83.9875) -> (173.6875, -96.9875)
  arc A284 (160.1875, -83.4875) -> (159.6875, -83.9875) centre (160.1875, -83.9875) ccw
  arc A285 (173.6875, -83.9875) -> (173.1875, -83.4875) centre (173.1875, -83.9875) ccw
  arc A286 (159.6875, -96.9875) -> (160.1875, -97.4875) centre (160.1875, -96.9875) ccw
  arc A287 (173.1875, -97.4875) -> (173.6875, -96.9875) centre (173.1875, -96.9875) ccw
  line L288 (179.2375, -83.4875) -> (192.2375, -83.4875)
  line L289 (179.2375, -97.4875) -> (192.2375, -97.4875)
  line L290 (178.7375, -83.9875) -> (178.7375, -96.9875)
  line L291 (192.7375, -83.9875) -> (192.7375, -96.9875)
  arc A288 (179.2375, -83.4875) -> (178.7375, -83.9875) centre (179.2375, -83.9875) ccw
  arc A289 (192.7375, -83.9875) -> (192.2375, -83.4875) centre (192.2375, -83.9875) ccw
  arc A290 (178.7375, -96.9875) -> (179.2375, -97.4875) centre (179.2375, -96.9875) ccw
  arc A291 (192.2375, -97.4875) -> (192.7375, -96.9875) centre (192.2375, -96.9875) ccw
  line L292 (198.2875, -83.4875) -> (211.2875, -83.4875)
  line L293 (198.2875, -97.4875) -> (211.2875, -97.4875)
  line L294 (197.7875, -83.9875) -> (197.7875, -96.9875)
  line L295 (211.7875, -83.9875) -> (211.7875, -96.9875)
  arc A292 (198.2875, -83.4875) -> (197.7875, -83.9875) centre (198.2875, -83.9875) ccw
  arc A293 (211.7875, -83.9875) -> (211.2875, -83.4875) centre (211.2875, -83.9875) ccw
  arc A294 (197.7875, -96.9875) -> (198.2875, -97.4875) centre (198.2875, -96.9875) ccw
  arc A295 (211.2875, -97.4875) -> (211.7875, -96.9875) centre (211.2875, -96.9875) ccw
  line L296 (217.3375, -83.4875) -> (230.3375, -83.4875)
  line L297 (217.3375, -97.4875) -> (230.3375, -97.4875)
  line L298 (216.8375, -83.9875) -> (216.8375, -96.9875)
  line L299 (230.8375, -83.9875) -> (230.8375, -96.9875)
  arc A296 (217.3375, -83.4875) -> (216.8375, -83.9875) centre (217.3375, -83.9875) ccw
  arc A297 (230.8375, -83.9875) -> (230.3375, -83.4875) centre (230.3375, -83.9875) ccw
  arc A298 (216.8375, -96.9875) -> (217.3375, -97.4875) centre (217.3375, -96.9875) ccw
  arc A299 (230.3375, -97.4875) -> (230.8375, -96.9875) centre (230.3375, -96.9875) ccw
  line L300 (243.5313, -83.4875) -> (256.5313, -83.4875)
  line L301 (243.5313, -97.4875) -> (256.5313, -97.4875)
  line L302 (243.0312, -83.9875) -> (243.0312, -96.9875)
  line L303 (257.0312, -83.9875) -> (257.0312, -96.9875)
  arc A300 (243.5313, -83.4875) -> (243.0313, -83.9875) centre (243.5313, -83.9875) ccw
  arc A301 (257.0312, -83.9875) -> (256.5312, -83.4875) centre (256.5312, -83.9875) ccw
  arc A302 (243.0313, -96.9875) -> (243.5313, -97.4875) centre (243.5313, -96.9875) ccw
  arc A303 (256.5312, -97.4875) -> (257.0312, -96.9875) centre (256.5312, -96.9875) ccw
  line L304 (274.4875, -88.25) -> (287.4875, -88.25)
  line L305 (274.4875, -102.25) -> (287.4875, -102.25)
  line L306 (273.9875, -88.75) -> (273.9875, -101.75)
  line L307 (287.9875, -88.75) -> (287.9875, -101.75)
  arc A304 (274.4875, -88.25) -> (273.9875, -88.75) centre (274.4875, -88.75) ccw
  arc A305 (287.9875, -88.75) -> (287.4875, -88.25) centre (287.4875, -88.75) ccw
  arc A306 (273.9875, -101.75) -> (274.4875, -102.25) centre (274.4875, -101.75) ccw
  arc A307 (287.4875, -102.25) -> (287.9875, -101.75) centre (287.4875, -101.75) ccw
  line L308 (3.025, -102.5375) -> (16.025, -102.5375)
  line L309 (3.025, -116.5375) -> (16.025, -116.5375)
  line L310 (2.525, -103.0375) -> (2.525, -116.0375)
  line L311 (16.525, -103.0375) -> (16.525, -116.0375)
  arc A308 (3.025, -102.5375) -> (2.525, -103.0375) centre (3.025, -103.0375) ccw
  arc A309 (16.525, -103.0375) -> (16.025, -102.5375) centre (16.025, -103.0375) ccw
  arc A310 (2.525, -116.0375) -> (3.025, -116.5375) centre (3.025, -116.0375) ccw
  arc A311 (16.025, -116.5375) -> (16.525, -116.0375) centre (16.025, -116.0375) ccw
  line L312 (22.075, -102.5375) -> (35.075, -102.5375)
  line L313 (22.075, -116.5375) -> (35.075, -116.5375)
  line L314 (21.575, -103.0375) -> (21.575, -116.0375)
  line L315 (35.575, -103.0375) -> (35.575, -116.0375)
  arc A312 (22.075, -102.5375) -> (21.575, -103.0375) centre (22.075, -103.0375) ccw
  arc A313 (35.575, -103.0375) -> (35.075, -102.5375) centre (35.075, -103.0375) ccw
  arc A314 (21.575, -116.0375) -> (22.075, -116.5375) centre (22.075, -116.0375) ccw
  arc A315 (35.075, -116.5375) -> (35.575, -116.0375) centre (35.075, -116.0375) ccw
  line L316 (41.125, -102.5375) -> (54.125, -102.5375)
  line L317 (41.125, -116.5375) -> (54.125, -116.5375)
  line L318 (40.625, -103.0375) -> (40.625, -116.0375)
  line L319 (54.625, -103.0375) -> (54.625, -116.0375)
  arc A316 (41.125, -102.5375) -> (40.625, -103.0375) centre (41.125, -103.0375) ccw
  arc A317 (54.625, -103.0375) -> (54.125, -102.5375) centre (54.125, -103.0375) ccw
  arc A318 (40.625, -116.0375) -> (41.125, -116.5375) centre (41.125, -116.0375) ccw
  arc A319 (54.125, -116.5375) -> (54.625, -116.0375) centre (54.125, -116.0375) ccw
  line L320 (60.175, -102.5375) -> (73.175, -102.5375)
  line L321 (60.175, -116.5375) -> (73.175, -116.5375)
  line L322 (59.675, -103.0375) -> (59.675, -116.0375)
  line L323 (73.675, -103.0375) -> (73.675, -116.0375)
  arc A320 (60.175, -102.5375) -> (59.675, -103.0375) centre (60.175, -103.0375) ccw
  arc A321 (73.675, -103.0375) -> (73.175, -102.5375) centre (73.175, -103.0375) ccw
  arc A322 (59.675, -116.0375) -> (60.175, -116.5375) centre (60.175, -116.0375) ccw
  arc A323 (73.175, -116.5375) -> (73.675, -116.0375) centre (73.175, -116.0375) ccw
  line L324 (126.85, -102.5375) -> (139.85, -102.5375)
  line L325 (126.85, -116.5375) -> (139.85, -116.5375)
  line L326 (126.35, -103.0375) -> (126.35, -116.0375)
  line L327 (140.35, -103.0375) -> (140.35, -116.0375)
  arc A324 (126.85, -102.5375) -> (126.35, -103.0375) centre (126.85, -103.0375) ccw
  arc A325 (140.35, -103.0375) -> (139.85, -102.5375) centre (139.85, -103.0375) ccw
  arc A326 (126.35, -116.0375) -> (126.85, -116.5375) centre (126.85, -116.0375) ccw
  arc A327 (139.85, -116.5375) -> (140.35, -116.0375) centre (139.85, -116.0375) ccw
  line L328 (82.725, -103.5375) -> (88.725, -103.5375)
  line L329 (82.725, -118.5375) -> (88.725, -118.5375)
  line L330 (82.225, -104.0375) -> (82.225, -118.0375)
  line L331 (89.225, -104.0375) -> (89.225, -118.0375)
  arc A328 (82.725, -103.5375) -> (82.225, -104.0375) centre (82.725, -104.0375) ccw
  arc A329 (89.225, -104.0375) -> (88.725, -103.5375) centre (88.725, -104.0375) ccw
  arc A330 (82.225, -118.0375) -> (82.725, -118.5375) centre (82.725, -118.0375) ccw
  arc A331 (88.725, -118.5375) -> (89.225, -118.0375) centre (88.725, -118.0375) ccw
  line L332 (177.975, -103.5375) -> (183.975, -103.5375)
  line L333 (177.975, -118.5375) -> (183.975, -118.5375)
  line L334 (177.475, -104.0375) -> (177.475, -118.0375)
  line L335 (184.475, -104.0375) -> (184.475, -118.0375)
  arc A332 (177.975, -103.5375) -> (177.475, -104.0375) centre (177.975, -104.0375) ccw
  arc A333 (184.475, -104.0375) -> (183.975, -103.5375) centre (183.975, -104.0375) ccw
  arc A334 (177.475, -118.0375) -> (177.975, -118.5375) centre (177.975, -118.0375) ccw
  arc A335 (183.975, -118.5375) -> (184.475, -118.0375) centre (183.975, -118.0375) ccw
  line L336 (193.525, -102.5375) -> (206.525, -102.5375)
  line L337 (193.525, -116.5375) -> (206.525, -116.5375)
  line L338 (193.025, -103.0375) -> (193.025, -116.0375)
  line L339 (207.025, -103.0375) -> (207.025, -116.0375)
  arc A336 (193.525, -102.5375) -> (193.025, -103.0375) centre (193.525, -103.0375) ccw
  arc A337 (207.025, -103.0375) -> (206.525, -102.5375) centre (206.525, -103.0375) ccw
  arc A338 (193.025, -116.0375) -> (193.525, -116.5375) centre (193.525, -116.0375) ccw
  arc A339 (206.525, -116.5375) -> (207.025, -116.0375) centre (206.525, -116.0375) ccw
  line L340 (212.575, -102.5375) -> (225.575, -102.5375)
  line L341 (212.575, -116.5375) -> (225.575, -116.5375)
  line L342 (212.075, -103.0375) -> (212.075, -116.0375)
  line L343 (226.075, -103.0375) -> (226.075, -116.0375)
  arc A340 (212.575, -102.5375) -> (212.075, -103.0375) centre (212.575, -103.0375) ccw
  arc A341 (226.075, -103.0375) -> (225.575, -102.5375) centre (225.575, -103.0375) ccw
  arc A342 (212.075, -116.0375) -> (212.575, -116.5375) centre (212.575, -116.0375) ccw
  arc A343 (225.575, -116.5375) -> (226.075, -116.0375) centre (225.575, -116.0375) ccw
  line L344 (231.625, -102.5375) -> (244.625, -102.5375)
  line L345 (231.625, -116.5375) -> (244.625, -116.5375)
  line L346 (231.125, -103.0375) -> (231.125, -116.0375)
  line L347 (245.125, -103.0375) -> (245.125, -116.0375)
  arc A344 (231.625, -102.5375) -> (231.125, -103.0375) centre (231.625, -103.0375) ccw
  arc A345 (245.125, -103.0375) -> (244.625, -102.5375) centre (244.625, -103.0375) ccw
  arc A346 (231.125, -116.0375) -> (231.625, -116.5375) centre (231.625, -116.0375) ccw
  arc A347 (244.625, -116.5375) -> (245.125, -116.0375) centre (244.625, -116.0375) ccw
  line L348 (255.4375, -107.3) -> (268.4375, -107.3)
  line L349 (255.4375, -121.3) -> (268.4375, -121.3)
  line L350 (254.9375, -107.8) -> (254.9375, -120.8)
  line L351 (268.9375, -107.8) -> (268.9375, -120.8)
  arc A348 (255.4375, -107.3) -> (254.9375, -107.8) centre (255.4375, -107.8) ccw
  arc A349 (268.9375, -107.8) -> (268.4375, -107.3) centre (268.4375, -107.8) ccw
  arc A350 (254.9375, -120.8) -> (255.4375, -121.3) centre (255.4375, -120.8) ccw
  arc A351 (268.4375, -121.3) -> (268.9375, -120.8) centre (268.4375, -120.8) ccw
  line L352 (274.4875, -107.3) -> (287.4875, -107.3)
  line L353 (274.4875, -121.3) -> (287.4875, -121.3)
  line L354 (273.9875, -107.8) -> (273.9875, -120.8)
  line L355 (287.9875, -107.8) -> (287.9875, -120.8)
  arc A352 (274.4875, -107.3) -> (273.9875, -107.8) centre (274.4875, -107.8) ccw
  arc A353 (287.9875, -107.8) -> (287.4875, -107.3) centre (287.4875, -107.8) ccw
  arc A354 (273.9875, -120.8) -> (274.4875, -121.3) centre (274.4875, -120.8) ccw
  arc A355 (287.4875, -121.3) -> (287.9875, -120.8) centre (287.4875, -120.8) ccw
  line L356 (293.5375, -107.3) -> (306.5375, -107.3)
  line L357 (293.5375, -121.3) -> (306.5375, -121.3)
  line L358 (293.0375, -107.8) -> (293.0375, -120.8)
  line L359 (307.0375, -107.8) -> (307.0375, -120.8)
  arc A356 (293.5375, -107.3) -> (293.0375, -107.8) centre (293.5375, -107.8) ccw
  arc A357 (307.0375, -107.8) -> (306.5375, -107.3) centre (306.5375, -107.8) ccw
  arc A358 (293.0375, -120.8) -> (293.5375, -121.3) centre (293.5375, -120.8) ccw
  arc A359 (306.5375, -121.3) -> (307.0375, -120.8) centre (306.5375, -120.8) ccw